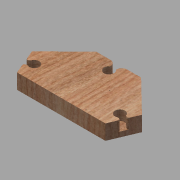
# Autodesk Inventor part: triangulo madera 2
Saved by Autodesk Inventor 2014 (Build 180170000, 170)
## iProperties
Created: 2016-10-24
Part Number: triangulo madera 2
Material: Wood (Birch)
Document SubType Name: Modeling
Designer: Cristian
Density: 0.55 g/cm^3
Appearance: Birch - Natural Polished
Author: Cristian
Autodesk Inventor part; units mm, degrees
ref_plane "YZ Plane" through (0, 0, 0) normal (1, 0, 0) x (0, 1, 0)
ref_plane "XZ Plane" through (0, 0, 0) normal (0, 1, 0) x (-1, 0, 0)
ref_plane "XY Plane" through (0, 0, 0) normal (0, 0, 1) x (1, 0, 0)
sketch "Sketch1" plane through (0, 0, 0) normal (0, 0, 1) x (1, 0, 0)
  line L0 (0, 0) -> (113, 0) construction
  line L1 (113, 0) -> (-113, 0) construction
  line L2 (0, 0) -> (0, 110) construction
  circle A0 centre (0, 110) radius 13
  circle A1 centre (-113, 0) radius 13
  circle A2 centre (113, 0) radius 13
  line L3 (0, 110) -> (-113, 0) construction
  line L4 (-113, 0) -> (0, 110) construction
  line L5 (113, 0) -> (0, 110) construction
  line L6 (-113, 0) -> (-113, 13) construction
  line L7 (113, 0) -> (113, 13) construction
  line L8 (0, 110) -> (13, 110) construction
  line L9 (0, 110) -> (-13, 110) construction
  line L10 (113, 0) -> (113, -13) construction
  line L11 (-113, 0) -> (-113, -13) construction
  line L12 (-113, 0) -> (-93, 0) construction
  line L13 (-113, 0) -> (-113, -20) construction
  line L14 (0, 110) -> (-14.3558, 123.9252) construction
  line L15 (-113, 0) -> (-127.3558, 13.9252) construction
  line L16 (-127.3558, 13.9252) -> (-14.3558, 123.9252) construction
  line L17 (-127.3558, 13.9252) -> (-109.442, 31.3634) construction
  line L18 (113, 0) -> (113, -20) construction
  line L19 (113, -20) -> (-113, -20) construction
  line L20 (-113, -20) -> (-88, -20) construction
  line L21 (-88, -20) -> (-109.442, 31.3634) construction
  line L22 (127.3558, 13.9252) -> (14.3558, 123.9252) construction
  line L23 (127.3558, 13.9252) -> (109.442, 31.3634) construction
  line L24 (113, -20) -> (88, -20) construction
  line L25 (88, -20) -> (109.442, 31.3634) construction
  line L26 (0, 110) -> (-28.6608, 110) construction
  line L27 (0, 110) -> (28.6608, 110) construction
  line L28 (-28.6608, 110) -> (-44.425, 94.6543) construction
  line L29 (-44.425, 94.6543) -> (44.425, 94.6543) construction
  line L30 (-109.442, 31.3634) -> (-44.425, 94.6543)
  line L31 (44.425, 94.6543) -> (109.442, 31.3634)
  line L32 (88, -20) -> (-88, -20)
  line L33 (-88, -20) -> (-109.442, 31.3634)
  line L34 (88, -20) -> (109.442, 31.3634)
  line L35 (-44.425, 94.6543) -> (44.425, 94.6543)
  dimension "d0" = 113
  dimension "d1" = 226
  dimension "d2" = 110
  dimension "d3" = 26
  dimension "d5" = 26
  dimension "d14" = 20
  dimension "d17" = 20
  dimension "d18" = 20
  dimension "d19" = 25
  dimension "d20" = 20
  dimension "d21" = 25
  dimension "d22" = 25
  dimension "d23" = 25
  dimension "d24" = 22
  constraints: 72 end point, 9 point on line, 8 horizontal, 7 vertical, 6 point on circle, 4 collinear, 3 centre point, 3 coincident, 2 symmetric about line, 1 parallel
  measures "d0" distance of L0.start L0.end
  measures "d1" distance of L0.end L1.end
  measures "d2" distance of L0.start L2.end
  measures "d3" diameter of A0
  measures "d5" diameter of A2
  measures "d14" distance of L3.end L13.end
  measures "d17" distance of L3.start L14.end
  measures "d18" distance of L3.end L15.end
  measures "d19" distance of L15.end L17.end
  measures "d20" distance of L5.start L18.end
  measures "d21" distance of L13.end L20.end
  measures "d22" distance of L22.start L23.end
  measures "d23" distance of L18.end L24.end
  measures "d24" distance of L26.end L28.end
extrude "Extrusion1" add sketch "Sketch1" along normal blind 30 contours L30 L35 L31 L34 L32 L33
sketch "Sketch2" plane through (0, 0, 30) normal (0, 0, 1) x (1, 0, 0)
  circle A0 centre (-85.3155, 11.5571) radius 2.5 projected
  circle A1 centre (-113, 0) radius 13 projected
  line L0 (-109.442, 31.3634) -> (-126.5339, 14.7252) projected
  arc A2 (-126.5339, 14.7252) -> (-113, -20) centre (-113, 0) ccw projected
  line L1 (-113, -20) -> (-88, -20) projected
  line L2 (-88, -20) -> (-95.5255, -1.9729) projected
  arc A3 (-93.9357, 1.9416) -> (-95.5255, -1.9729) centre (-92.7571, -0.8172) ccw projected
  arc A4 (-90.1342, 2.7946) -> (-93.9357, 1.9416) centre (-89.7305, -7.9015) ccw projected
  arc A5 (-90.1342, 2.7946) -> (-94.934, 14.2926) centre (-85.3155, 11.5571) ccw projected
  arc A6 (-98.2137, 12.1895) -> (-94.934, 14.2926) centre (-102.2552, 22.1009) ccw projected
  arc A7 (-102.1149, 13.8117) -> (-98.2137, 12.1895) centre (-99.3465, 14.9674) ccw projected
  line L3 (-102.1149, 13.8117) -> (-109.442, 31.3634) projected
  circle A8 centre (0, 75) radius 2.5 projected
  circle A9 centre (0, 110) radius 13 projected
  line L4 (44.425, 94.6543) -> (17.7482, 123) projected
  arc A10 (17.7482, 123) -> (-17.7482, 123) centre (0, 110) ccw projected
  line L5 (-17.7482, 123) -> (-44.425, 94.6543) projected
  line L6 (-44.425, 94.6543) -> (-16.0004, 94.6543) projected
  arc A11 (-6.0005, 84.6098) -> (-16.0004, 94.6543) centre (-16.0004, 84.6543) ccw projected
  arc A12 (-6.0352, 82.9735) -> (-6.0005, 84.6098) centre (-54.7865, 84.8272) ccw projected
  arc A13 (-6.0352, 82.9735) -> (6.0352, 82.9735) centre (0, 75) ccw projected
  arc A14 (6.0005, 84.6098) -> (6.0352, 82.9735) centre (54.7865, 84.8272) ccw projected
  arc A15 (16.0004, 94.6543) -> (6.0005, 84.6098) centre (16.0004, 84.6543) ccw projected
  line L7 (16.0004, 94.6543) -> (44.425, 94.6543) projected
  circle A16 centre (85.3155, 11.5571) radius 2.5 projected
  circle A17 centre (113, 0) radius 13 projected
  line L8 (88, -20) -> (113, -19.9918) projected
  arc A18 (113, -19.9918) -> (126.9449, 14.3252) centre (113, 0) ccw projected
  line L9 (126.9449, 14.3252) -> (109.442, 31.3634) projected
  line L10 (109.442, 31.3634) -> (102.1149, 13.8117) projected
  arc A19 (98.2137, 12.1895) -> (102.1149, 13.8117) centre (99.3465, 14.9674) ccw projected
  arc A20 (94.934, 14.2926) -> (98.2137, 12.1895) centre (102.2552, 22.1009) ccw projected
  arc A21 (94.934, 14.2926) -> (90.1342, 2.7946) centre (85.3155, 11.5571) ccw projected
  arc A22 (93.9357, 1.9416) -> (90.1342, 2.7946) centre (89.7305, -7.9015) ccw projected
  arc A23 (95.5255, -1.9729) -> (93.9357, 1.9416) centre (92.7571, -0.8172) ccw projected
  line L11 (95.5255, -1.9729) -> (88, -20) projected
  arc A24 (-6.0005, 84.6098) -> (-16.0004, 94.6543) centre (-16.0004, 84.6543) ccw projected
  point P0 (0, 0)
extrude "Extrusion2" cut sketch "Sketch2" against normal blind 20 contours A0 | L3 A7 A6 A5 A4 A3 L2 L1 A2 L0 | A8 | L7 A15 A14 A13 A12 A11 L6 L5 A10 L4 | A16 | L11 A23 A22 A21 A20 A19 L10 L9 A18 L8
body "Solid1"
